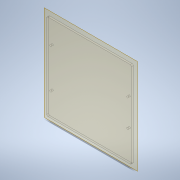
# Autodesk Inventor part: Lid
Saved by Autodesk Inventor 2022 (Build 260153000, 153)
## iProperties
Created: 2022-01-15
Part Number: Lid
Material: Polycarbonate, Clear
Document SubType Name: Modeling
Designer: siwat
Density: 1.2 g/cm^3
Appearance: Polycarbonate - Clear
VLDS_Profile: Default Part
VLDS_TimeStamp: 2022-02-27
VLDS_FailCnt: 3
VLDS_AcceptCnt: 0
Author: siwat
Autodesk Inventor part; units mm, degrees
ref_plane "YZ Plane" through (0, 0, 0) normal (1, 0, 0) x (0, 1, 0)
ref_plane "XZ Plane" through (0, 0, 0) normal (0, 1, 0) x (-1, 0, 0)
ref_plane "XY Plane" through (0, 0, 0) normal (0, 0, 1) x (1, 0, 0)
ref_plane "Work Plane1" through (0, 0, 0) normal (0, 0, 1) x (1, 0, 0)
sketch "Sketch1" plane through (0, 0, 0) normal (0, 0, 1) x (1, 0, 0)
  line L0 (71.2978, -72.4006) -> (-71.2977, -72.4006)
  line L1 (-71.2977, -72.4006) -> (-71.2977, 72.4006)
  line L2 (-71.2977, 72.4006) -> (71.2978, 72.4006)
  line L3 (71.2978, 72.4006) -> (71.2978, -72.4006)
  point P0 (0, 0)
  constraints: 8 end point, 2 parallel, 1 horizontal, 1 perpendicular
extrude "Extrusion1" add sketch "Sketch1" along normal blind 3
fillet "Fillet1" radius 2 4 edges at (-71.2977, 72.4006, 1.5) (-71.2977, -72.4006, 1.5) (71.2978, -72.4006, 1.5) (71.2978, 72.4006, 1.5)
sketch "Sketch2" plane through (0, 0, 3) normal (0, 0, 1) x (1, 0, 0)
  circle A0 centre (-64.7963, 32.8982) radius 1.5
  circle A1 centre (-64.7151, -33.0663) radius 1.5
  circle A2 centre (64.7357, -22.905) radius 1.5
  circle A3 centre (64.6752, 23.0253) radius 1.5
  point P0 (0, 0)
  dimension "d3" = 3
  dimension "d4" = 3
  dimension "d5" = 3
  dimension "d6" = 3
  constraints: 4 centre point
  measures "d3" diameter of A0
  measures "d4" diameter of A1
  measures "d5" diameter of A2
  measures "d6" diameter of A3
extrude "Extrusion2" cut sketch "Sketch2" against normal through all
body "Solid1"
